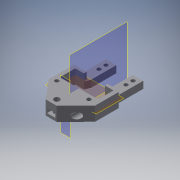
# Autodesk Inventor part: 30_Cube_Z_Focus_Drylin_NEMA_slide
Saved by Autodesk Inventor 2019.4 (Build 234330000, 330)
## iProperties
Created: 2021-04-25
Part Number: 30_Cube_Z_Focus_Drylin_NEMA_slide
Material: Generic
Document SubType Name: Modeling
Designer: diederichbenedict
Density: 1 g/cm^3
Appearance: Default
Author: diederichbenedict
Autodesk Inventor part; units mm, degrees
ref_plane "YZ Plane" through (0, 0, 0) normal (1, 0, 0) x (0, 1, 0)
ref_plane "Work Plane1" through (26.5, 0, 0) normal (0, 0, -1) x (-1, 0, 0)
sketch "Sketch1" plane through (-19.3, 0, 0) normal (0, 0, 1) x (1, 0, 0)
  circle A0 centre (2.9, -26.2) radius 1.75 projected
  circle A1 centre (2.9, -6.2) radius 1.75 projected
  circle A2 centre (22.9, -26.2) radius 1.75 projected
  circle A3 centre (22.9, -6.2) radius 1.75 projected
  line L0 (0.3744, -33.9) -> (0.3744, 2.1) construction
  line L1 (25.8, 0) -> (25.8, -32.4) construction
  line L2 (-0.6, 0) -> (-0.6, -32.4) construction
  line L3 (19.3, -32.4) -> (25.8, -32.4) construction
  line L4 (25.8, 0) -> (25.8, -32.4) construction
  line L5 (19.3, 0) -> (25.8, 0) construction
  line L6 (19.3, 0) -> (19.3, -32.4) construction
  circle A4 centre (22.9, -6.2) radius 1.75 construction
  circle A5 centre (22.9, -26.2) radius 1.75 construction
  line L7 (0, -32.4) -> (6.5, -32.4) construction
  line L8 (6.5, 0) -> (6.5, -32.4) construction
  line L9 (0, 0) -> (6.5, 0) construction
  line L10 (0, 0) -> (0, -32.4) construction
  circle A6 centre (2.9, -6.2) radius 1.75 construction
  circle A7 centre (2.9, -26.2) radius 1.75 construction
  line L11 (29.4, -10) -> (-3.6, -10)
  line L12 (-3.6, -10) -> (-3.6, 0)
  line L13 (-3.6, 0) -> (29.4, 0)
  line L14 (29.4, 0) -> (29.4, -10)
  circle A8 centre (22.9, -26.2) radius 2.25
  circle A9 centre (22.9, -6.2) radius 2.25
  circle A10 centre (2.9, -6.2) radius 2.25
  circle A11 centre (2.9, -26.2) radius 2.25
  line L15 (26.4, 0) -> (26.4, -32.4) projected
  dimension "d1" = 3
  dimension "d2" = 0.5
  dimension "d3" = 0.5
  dimension "d4" = 0.5
  dimension "d5" = 0.5
  dimension "d19" = 3
  dimension "d32" = 10
  constraints: 8 end point, 4 centre point, 2 vertical, 1 horizontal, 1 parallel, 5 other
  measures "d1" distance between parallel lines of L2 L12
  measures "d2" radial gap between concentric circles of A2 A8
  measures "d3" radial gap between concentric circles of A3 A9
  measures "d4" radial gap between concentric circles of A1 A10
  measures "d5" radial gap between concentric circles of A0 A11
  measures "d19" distance between parallel lines of L14 L15
extrude "Extrusion1" add sketch "Sketch1" along normal blind 5 contours L11 L15 L13 L14 | L11 L12 L13 L15
sketch "Sketch2" plane through (-19.3, 0, 0) normal (0, 0, -1) x (-1, 0, 0)
  circle A0 centre (-2.9, -6.2) radius 2.25 projected
  circle A1 centre (-22.9, -6.2) radius 2.25 projected
  line L0 (3.6, -10) -> (-29.4, -10) projected
  line L1 (-29.4, -10) -> (-29.4, 0) projected
  line L2 (-29.4, 0) -> (3.6, 0) projected
  line L3 (3.6, 0) -> (3.6, -10) projected
  line L4 (3.6, -10) -> (3.6, 0) projected
  line L5 (3.6, 0) -> (0.8, 0)
  line L6 (0.8, 0) -> (0.8, -10)
  line L7 (0.8, -10) -> (3.6, -10)
  line L8 (3.6, -10) -> (3.6, 0)
  line L9 (-29.4, -10) -> (3.6, -10) projected
  line L10 (-29.4, 0) -> (-26.6, 0)
  line L11 (-26.6, 0) -> (-26.6, -10)
  line L12 (-26.6, -10) -> (-29.4, -10)
  line L13 (-29.4, -10) -> (-29.4, 0)
  point P0 (-19.3, 0)
  dimension "d8" = 2.8
  dimension "d9" = 2.8
  dimension "d10" = 0
  constraints: 16 end point, 4 parallel, 3 point on line, 2 horizontal, 2 perpendicular
  measures "d8" distance of L7.end L6.end
  measures "d9" distance of L11.end L12.end
  measures "d10" distance between parallel lines of L2 L10
extrude "Extrusion2" add sketch "Sketch2" along normal blind 12 contours L0 L6 L2 L3 | L0 L1 L2 L11
sketch "Sketch3" plane through (-19.3, 0, -12) normal (0, 0, -1) x (-1, 0, 0)
  line L0 (-29.4, 0) -> (-29.4, -10) projected
  line L1 (-29.4, -10) -> (-26.6, -10) projected
  line L2 (-26.6, -10) -> (-26.6, 0) projected
  line L3 (-26.6, 0) -> (-29.4, 0) projected
  line L4 (3.6, -10) -> (3.6, 0) projected
  line L5 (3.6, 0) -> (0.8, 0) projected
  line L6 (0.8, 0) -> (0.8, -10) projected
  line L7 (-18.8691, 0.2794) -> (-18.8691, -79.7206) construction
  line L8 (-8.1725, 0.2794) -> (-8.1725, -79.7206) construction
  line L9 (-29.4, 0) -> (3.6, 0) construction
  line L10 (3.6, -10) -> (-29.4, -10) projected
  line L11 (-29.4, 0) -> (-20.4, 0)
  line L12 (-20.4, 0) -> (-20.4, -10)
  line L13 (-20.4, -10) -> (-29.4, -10)
  line L14 (-29.4, -10) -> (-29.4, 0)
  line L15 (3.6, 0) -> (3.6, -10) projected
  line L16 (3.6, 0) -> (-5.4, 0)
  line L17 (-5.4, 0) -> (-5.4, -10)
  line L18 (-5.4, -10) -> (3.6, -10)
  line L19 (3.6, -10) -> (3.6, 0)
  line L20 (0.8, -10) -> (3.6, -10) projected
  point P0 (-19.3, 0)
  dimension "d13" = 9
  dimension "d14" = 9
  constraints: 16 end point, 4 parallel, 2 horizontal, 2 perpendicular, 2 point on line
  measures "d13" distance of L12.end L13.end
  measures "d14" distance of L18.end L17.end
extrude "Extrusion3" add sketch "Sketch3" along normal blind 1 and the other way blind 1
ref_plane "Work Plane2" through (-22.9, -4, 5) normal (0, 1, 0) x (1, 0, 0)
sketch "Sketch4" plane through (-22.9, -10, 5) normal (0, 1, 0) x (1, 0, 0)
  line L0 (0, 0) -> (0, 18) projected
  line L1 (33, 0) -> (0, 0) projected
  line L2 (33, 0) -> (33, 18) projected
  line L3 (24, 18) -> (33, 18) projected
  line L4 (24, 18) -> (24, 16) projected
  line L5 (30.2, 16) -> (24, 16) projected
  line L6 (30.2, 5) -> (30.2, 16) projected
  line L7 (2.8, 5) -> (30.2, 5) projected
  line L8 (2.8, 5) -> (2.8, 16) projected
  line L9 (9, 16) -> (2.8, 16) projected
  line L10 (9, 16) -> (9, 18) projected
  line L11 (0, 18) -> (9, 18) projected
  line L12 (32.9002, 18.2) -> (30.3433, 20.7569) construction
  line L13 (-0.4956, 21.98) -> (-4.2756, 18.2) construction
  line L14 (34.2709, 21.1536) -> (36.398, 19.0265) construction
  line L15 (30.3433, 26.08) -> (30.3433, 18.1) construction
  line L16 (21.9706, 26.08) -> (21.9706, 18.1) construction
  line L17 (11.0029, 26.08) -> (11.0029, 18.1) construction
  line L18 (2.6055, 26.08) -> (2.6055, 20.7569) construction
  line L19 (24, 18) -> (33, 18) projected
  line L20 (31.5357, 18) -> (29.8433, 19.6923)
  line L21 (29.8433, 19.6923) -> (22.4706, 19.6923)
  line L22 (22.4706, 19.6923) -> (24, 16)
  line L23 (29.8433, 19.6923) -> (29.8433, 37.6831)
  line L24 (22.4706, 19.6923) -> (29.8433, 19.6923)
  line L25 (29.8433, 19.6923) -> (29.8433, 37.6831)
  line L26 (29.8433, 37.6831) -> (22.4706, 37.6831)
  line L27 (22.4706, 37.6831) -> (22.4706, 19.6923)
  point P0 (22.9, 5)
  dimension "d21" = 157.5
  dimension "d22" = 0.5
  dimension "d23" = 0.5
  constraints: 16 end point, 4 parallel, 1 horizontal, 1 perpendicular, 1 point on line, 1 vertical
  measures "d21" angle of L4 L22
  measures "d22" distance from line of L21.end L16
  measures "d23" distance between parallel lines of L15 L23
extrude "Extrusion4" add sketch "Sketch4" along normal blind 5
ref_plane "Work Plane3" through (-6.4, -10, 5) normal (-1, 0, 0) x (0, 0, 1)
mirror "Mirror1" about plane through (-6.4, -10, 5) normal (-1, 0, 0) of "Extrusion4"
chamfer "Chamfer2" distance 1 angle 45 4 edges at (9.3678, -10, -13) (-22.1678, -10, -13) (-17.6678, -5, -13) (4.8678, -5, -13)
sketch "Sketch5" plane through (-22.9, -5, 5) normal (0, 1, 0) x (1, 0, 0)
  line L0 (24, 19) -> (24, 16) projected
  line L1 (30.5357, 19) -> (24, 19) projected
  line L2 (30.5357, 19) -> (29.8433, 19.6923) projected
  line L3 (29.8433, 19.6923) -> (29.8433, 37.6831) projected
  line L4 (29.8433, 37.6831) -> (22.4706, 37.6831) projected
  line L5 (22.4706, 37.6831) -> (22.4706, 19.6923) projected
  line L6 (22.4706, 19.6923) -> (24, 16) projected
  line L7 (9, 19) -> (2.4643, 19) projected
  line L8 (9, 16) -> (9, 19) projected
  line L9 (10.5294, 19.6923) -> (9, 16) projected
  line L10 (10.5294, 37.6831) -> (10.5294, 19.6923) projected
  line L11 (3.1567, 37.6831) -> (10.5294, 37.6831) projected
  line L12 (3.1567, 19.6923) -> (3.1567, 37.6831) projected
  line L13 (2.4643, 19) -> (3.1567, 19.6923) projected
  circle A0 centre (26.1569, 33.9967) radius 3.6864
  circle A1 centre (6.843, 33.9967) radius 3.6864
  circle A2 centre (26.1569, 33.9967) radius 1.4
  circle A3 centre (6.843, 33.9967) radius 1.4
  circle A4 centre (26.1569, 28.9967) radius 1.4
  circle A5 centre (6.843, 28.9967) radius 1.4
  point P0 (22.9, 5)
  dimension "d33" = 2.8
  dimension "d34" = 2.8
  dimension "d37" = 2.8
  dimension "d38" = 2.8
  dimension "d39" = 5
  dimension "d40" = 5
  constraints: 6 centre point, 6 tangent, 2 coincident
  measures "d33" diameter of A2
  measures "d34" diameter of A3
  measures "d37" diameter of A4
  measures "d38" diameter of A5
  measures "d39" distance of A0.centre A4.centre
  measures "d40" distance of A5.centre A1.centre
extrude "Extrusion5" cut sketch "Sketch5" against normal through all contours A4 A0 | A0 A4 | A5 A1 | A1 A5 | A2 | A3 picked at (26.2031, 30.3641) picked at (26.0901, 28.5093) picked at (6.8892, 30.3641) picked at (6.7762, 28.5093)
sketch "Sketch6" plane through (-22.9, -10, 5) normal (0, 1, 0) x (1, 0, 0)
  line L0 (0, 0) -> (0, 18) projected
  line L1 (33, 0) -> (0, 0) projected
  line L2 (33, 0) -> (33, 18) projected
  line L3 (24, 18) -> (33, 18) projected
  line L4 (24, 18) -> (24, 16) projected
  line L5 (30.2, 16) -> (24, 16) projected
  line L6 (30.2, 5) -> (30.2, 16) projected
  line L7 (2.8, 5) -> (30.2, 5) projected
  line L8 (2.8, 5) -> (2.8, 16) projected
  line L9 (9, 16) -> (2.8, 16) projected
  line L10 (9, 16) -> (9, 18) projected
  line L11 (0, 18) -> (9, 18) projected
  circle A0 centre (15.4444, -9.8) radius 1.1933 projected
  line L12 (0, 0) -> (11.4444, -13.8)
  line L13 (11.4444, -13.8) -> (19.4444, -13.8)
  line L14 (33, 0) -> (33, 18) projected
  line L15 (19.4444, -13.8) -> (33, 0)
  circle A1 centre (15.4444, -9.8) radius 2
  point P0 (22.9, 5)
  dimension "d41" = 4
  dimension "d42" = 4
  dimension "d43" = 4
  dimension "d44" = 4
  constraints: 6 end point, 1 centre point, 1 coincident, 1 horizontal
  measures "d41" distance from line of L13 A0.centre
  measures "d42" horizontal distance of L12.end A0.centre
  measures "d43" horizontal distance of L13.end A0.centre
  measures "d44" diameter of A1
ref_plane "Work Plane4" through (-24.55, -10, -34.5672) normal (0, -1, 0) x (1, 0, 0)
extrude "Extrusion6" add sketch "Sketch6" along normal up to surface (10 mm away) contours L1 L15 L13 L12
ref_plane "Work Plane5" through (-19.3, -32.4, 0) normal (0, 0, 1) x (1, 0, 0)
sketch "Sketch7" plane through (-19.3, 0, 5) normal (0, 0, 1) x (1, 0, 0)
  circle A0 centre (2.9, -6.2) radius 1.5 projected
  circle A1 centre (22.9, -6.2) radius 1.25 projected
  circle A2 centre (2.9, -6.2) radius 2.25
  circle A3 centre (22.9, -6.2) radius 2.25
  point P0 (19.3, 0)
  dimension "d47" = 4.5
  dimension "d48" = 4.5
  constraints: 2 centre point, 2 coincident
  measures "d47" diameter of A2
  measures "d48" diameter of A3
extrude "Extrusion7" cut sketch "Sketch7" against normal up to surface (5 mm away) contours A0 | A1 | A2 | A3
sketch "Sketch8" plane through (-11.4556, -10, 18.8) normal (0, 0, 1) x (1, 0, 0)
  line L0 (0, 0) -> (8, 0) projected
  line L1 (8, 0) -> (8, 10) projected
  line L2 (0, 0) -> (0, 10) projected
  line L3 (2.5, 13.1294) -> (2.5, 10.1294)
  line L4 (5.5, 13.1294) -> (5.5, 10.1294)
  line L5 (1, 5) -> (7, 5)
  line L6 (7, 5) -> (7, 2)
  line L7 (7, 2) -> (1, 2)
  line L8 (1, 2) -> (1, 5)
  line L9 (1, 5) -> (7, 2) construction
  line L10 (7, 5) -> (1, 2) construction
  line L11 (8, 10) -> (0, 10) projected
  point P0 (11.4556, 10)
  point P1 (4, 3.5)
  dimension "d51" = 6
  dimension "d52" = 3
  constraints: 16 end point, 2 midpoint, 2 parallel, 2 vertical, 1 horizontal, 1 perpendicular, 4 other
  measures "d51" distance of L6.end L7.end
  measures "d52" distance of L5.end L6.end
extrude "Extrusion8" cut sketch "Sketch8" against normal blind 8 contours L5 L6 L7 L8
sketch "Sketch9" plane through (-19.3, 0, 5) normal (0, 0, 1) x (1, 0, 0)
  circle A0 centre (2.9, -6.2) radius 1.75 projected
  circle A1 centre (22.9, -6.2) radius 1.75 projected
  circle A2 centre (2.9, -6.2) radius 2.25 projected
  circle A3 centre (22.9, -6.2) radius 2.25 projected
  point P0 (19.3, 0)
extrude "Extrusion9" cut sketch "Sketch9" along normal through all contours A0 | A1 | A2 | A3
chamfer "Chamfer3" distance 1 angle 45 2 edges at (10.1, -4.5, -13) (-22.9, -4.5, -13)
sketch "Sketch10" plane through (-20.1, 0, 0) normal (0, 1, 0) x (1, 0, 0)
  circle A0 centre (1.1444, -3.3) radius 1.25 projected
  circle A1 centre (24.1444, -3.3) radius 1.25 projected
  circle A2 centre (1.1444, -3.3) radius 1.45
  circle A3 centre (24.1444, -3.3) radius 1.45
  point P0 (20.1, 0)
  dimension "d60" = 2.9
  dimension "d61" = 2.9
  constraints: 2 centre point, 2 coincident
  measures "d60" diameter of A2
  measures "d61" diameter of A3
extrude "Extrusion10" cut sketch "Sketch10" against normal through all contours A0 | A1 | A2 | A3
body "Solid1"
